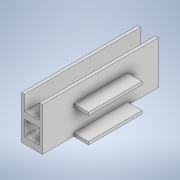
# Autodesk Inventor part: fuselage_tail_interface_v2
Saved by Autodesk Inventor 2021 (Build 250183000, 183)
## iProperties
Created: 2020-11-20
Part Number: fuselage_tail_interface_v2
Material: Generic
Document SubType Name: Modeling
Designer: Paco
Density: 1 g/cm^3
Appearance: Default
Author: Paco
Autodesk Inventor part; units mm, degrees
ref_plane "YZ Plane" through (0, 0, 0) normal (1, 0, 0) x (0, 1, 0)
ref_plane "XZ Plane" through (0, 0, 0) normal (0, 1, 0) x (-1, 0, 0)
ref_plane "XY Plane" through (0, 0, 0) normal (0, 0, 1) x (1, 0, 0)
sketch "Sketch1" plane through (0, 0, 0) normal (0, 0, 1) x (1, 0, 0)
  line L0 (-36.8287, 15.6534) -> (-26.8287, 15.6534)
  line L1 (-26.8287, 15.6534) -> (-26.8287, 5.6534)
  line L2 (-26.8287, 5.6534) -> (-36.8287, 5.6534)
  line L3 (-36.8287, 5.6534) -> (-36.8287, 15.6534)
  line L4 (-31.8287, 15.6534) -> (-31.8287, 5.6534) construction
  line L5 (-31.8287, 20.1534) -> (-48.8287, 20.1534)
  line L6 (-48.8287, 20.1534) -> (-48.8287, 18.1534)
  line L7 (-48.8287, 18.1534) -> (-38.8287, 18.1534)
  line L8 (-38.8287, 18.1534) -> (-38.8287, 3.1534)
  line L9 (-38.8287, 3.1534) -> (-48.8287, 3.1534)
  line L10 (-48.8287, 3.1534) -> (-48.8287, 1.1534)
  line L11 (-48.8287, 1.1534) -> (-31.8287, 1.1534)
  line L12 (-36.8287, 10.6534) -> (-26.8287, 10.6534) construction
  line L13 (-31.8287, 20.1534) -> (-14.8287, 20.1534)
  line L14 (-14.8287, 20.1534) -> (-14.8287, 18.1534)
  line L15 (-14.8287, 18.1534) -> (-24.8287, 18.1534)
  line L16 (-24.8287, 18.1534) -> (-24.8287, 3.1534)
  line L17 (-24.8287, 3.1534) -> (-14.8287, 3.1534)
  line L18 (-14.8287, 3.1534) -> (-14.8287, 1.1534)
  line L19 (-14.8287, 1.1534) -> (-31.8287, 1.1534)
  dimension "d3" = 10
  dimension "d4" = 10
  dimension "d5" = 15
  dimension "d6" = 2
  dimension "d7" = 2
  dimension "d8" = 4.5
  dimension "d9" = 4.5
  dimension "d10" = 2
  dimension "d11" = 10
  dimension "d13" = 17
  dimension "d14" = 17
  constraints: 40 end point, 6 perpendicular, 6 symmetric about line, 4 midpoint, 4 point on line, 2 horizontal, 2 parallel
  measures "d3" distance of L0.start L0.end
  measures "d4" distance of L0.end L1.end
  measures "d5" distance between parallel lines of L9 L7
  measures "d6" distance of L5.end L6.end
  measures "d7" distance of L9.end L10.end
  measures "d8" distance between parallel lines of L0 L5
  measures "d9" distance between parallel lines of L11 L2
  measures "d10" distance between parallel lines of L8 L3
  measures "d11" distance of L6.end L7.end
  measures "d13" distance of L5.start L5.end
  measures "d14" distance of L10.end L11.end
extrude "Extrusion1" add sketch "Sketch1" along normal blind 36
sketch "Sketch2" plane through (0, 0, 36) normal (0, 0, 1) x (1, 0, 0)
  line L0 (-36.8287, 5.6534) -> (-36.8287, 15.6534) projected
  line L1 (-26.8287, 5.6534) -> (-36.8287, 5.6534) projected
  line L2 (-36.8287, 15.6534) -> (-26.8287, 15.6534)
  line L3 (-26.8287, 15.6534) -> (-26.8287, 5.6534)
  line L4 (-26.8287, 5.6534) -> (-36.8287, 5.6534)
  line L5 (-36.8287, 5.6534) -> (-36.8287, 15.6534)
  line L6 (-38.8287, 20.1534) -> (-24.8287, 20.1534)
  line L7 (-24.8287, 20.1534) -> (-24.8287, 1.1534)
  line L8 (-24.8287, 1.1534) -> (-38.8287, 1.1534)
  line L9 (-38.8287, 1.1534) -> (-38.8287, 20.1534)
  line L10 (-14.8287, 20.1534) -> (-48.8287, 20.1534) projected
  point P0 (0, 0)
  dimension "d17" = 14
  dimension "d19" = 4.5
  dimension "d20" = 4.5
  dimension "d21" = 2
  dimension "d22" = 2
  constraints: 16 end point, 4 parallel, 2 horizontal, 2 perpendicular, 1 collinear
  measures "d17" distance of L6.start L6.end
  measures "d19" distance between parallel lines of L2 L6
  measures "d20" distance between parallel lines of L8 L1
  measures "d21" distance between parallel lines of L9 L0
  measures "d22" distance between parallel lines of L7 L3
extrude "Extrusion2" add sketch "Sketch2" along normal blind 21
sketch "Sketch3" plane through (0, 0, 0) normal (0, 0, -1) x (-1, 0, 0)
  line L0 (26.8287, 5.6534) -> (26.8287, 15.6534)
  line L1 (36.8287, 5.6534) -> (26.8287, 5.6534)
  line L2 (26.8287, 15.6534) -> (36.8287, 15.6534)
  line L3 (36.8287, 15.6534) -> (36.8287, 5.6534)
  line L4 (36.8287, 5.6534) -> (26.8287, 5.6534)
  line L5 (26.8287, 5.6534) -> (26.8287, 15.6534)
  line L6 (24.8287, 20.1534) -> (38.8287, 20.1534)
  line L7 (38.8287, 20.1534) -> (38.8287, 1.1534)
  line L8 (38.8287, 1.1534) -> (24.8287, 1.1534)
  line L9 (24.8287, 1.1534) -> (24.8287, 20.1534)
  line L10 (49.3332, 20.1534) -> (15.3332, 20.1534)
  line L11 (36.8287, 15.6534) -> (26.8287, 15.6534) projected
  line L12 (26.8287, 5.6534) -> (36.8287, 5.6534) projected
  line L13 (36.8287, 5.6534) -> (36.8287, 15.6534) projected
  line L14 (26.8287, 15.6534) -> (26.8287, 5.6534) projected
  line L15 (14.8287, 20.1534) -> (48.8287, 20.1534) projected
  point P0 (0, 0)
  dimension "d25" = 14
  dimension "d26" = 4.5
  dimension "d27" = 4.5
  dimension "d28" = 2
  dimension "d29" = 2
  constraints: 22 end point, 6 collinear, 4 parallel, 2 horizontal, 2 perpendicular
  measures "d25" distance of L6.start L6.end
  measures "d26" distance between parallel lines of L2 L6
  measures "d27" distance between parallel lines of L8 L1
  measures "d28" distance between parallel lines of L9 L0
  measures "d29" distance between parallel lines of L7 L3
extrude "Extrusion3" add sketch "Sketch3" along normal blind 21
sketch "Sketch4" plane through (0, 0, 57) normal (0, 0, 1) x (1, 0, 0)
  line L0 (-38.8287, 20.1534) -> (-48.8287, 20.1534) projected
  line L1 (-38.8287, 20.1534) -> (-38.8287, 30.1534)
  line L2 (-38.8287, 30.1534) -> (-36.8287, 30.1534)
  line L3 (-36.8287, 30.1534) -> (-36.8287, 20.1534)
  line L4 (-36.8287, 20.1534) -> (-26.8287, 20.1534)
  line L5 (-24.8287, 20.1534) -> (-38.8287, 20.1534) projected
  line L6 (-26.8287, 30.1534) -> (-24.8287, 30.1534)
  line L7 (-24.8287, 30.1534) -> (-24.8287, 20.1534)
  line L8 (-26.8287, 30.1534) -> (-26.8287, 20.1534)
  line L9 (-38.8287, 20.1534) -> (-38.8287, 1.1534) projected
  line L10 (-38.8287, 20.1534) -> (-36.8287, 20.1534)
  line L11 (-14.8287, 20.1534) -> (-24.8287, 20.1534) projected
  line L12 (-24.8287, 20.1534) -> (-26.8287, 20.1534)
  point P0 (0, 0)
  dimension "d32" = 2
  dimension "d33" = 2
  dimension "d34" = 10
  constraints: 18 end point, 3 perpendicular, 3 point on line, 2 collinear, 2 vertical
  measures "d32" distance of L1.end L2.end
  measures "d33" distance of L6.start L6.end
  measures "d34" distance of L6.end L5.start
extrude "Extrusion4" add sketch "Sketch4" against normal up to surface (78 mm away)
equation "\"d4\" = d3"
equation "\"d7\" = d6"
equation "\"d8\" = d9"
equation "\"d14\" = d13"
equation "\"d19\" = d20"
equation "\"d21\" = d22"
equation "\"d26\" = d27"
equation "\"d28\" = d29"
body "Solid1"
